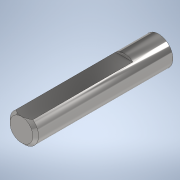
# Autodesk Inventor part: Stepper Motor Shaft
Saved by Autodesk Inventor 2022 (Build 260153000, 153)
## iProperties
Created: 2021-07-23
Part Number: Stepper Motor Shaft
Material: Generic
Document SubType Name: Modeling
Designer: John
Density: 1 g/cm^3
Appearance: Steel - Polished
Author: John
Autodesk Inventor part; units mm, degrees
ref_plane "YZ Plane" through (0, 0, 0) normal (1, 0, 0) x (0, 1, 0)
ref_plane "XZ Plane" through (0, 0, 0) normal (0, 1, 0) x (-1, 0, 0)
ref_plane "XY Plane" through (0, 0, 0) normal (0, 0, 1) x (1, 0, 0)
sketch "Sketch1" plane through (0, 0, 0) normal (0, 0, 1) x (1, 0, 0)
  circle A0 centre (0, 0) radius 2.5
  line L0 (-1.5, 2) -> (1.5, 2)
  dimension "d0" = 5
  constraints: 2 end point, 2 point on circle, 1 centre point, 1 coincident, 1 horizontal
  measures "d0" diameter of A0
sketch "Sketch1 outline for Extrusion1" plane through (0, 0, 0) normal (0, 0, 1) x (1, 0, 0)
  line L0 (1.5, 2) -> (-1.5, 2)
  arc A0 (-1.5, 2) -> (1.5, 2) centre (0, 0) ccw
extrude "Extrusion1" add sketch "Sketch1 outline for Extrusion1" along normal blind 24
sketch "Sketch2" plane through (0, 0, 0) normal (0, 0, -1) x (-1, 0, 0)
  line L0 (-1.5, 2) -> (1.5, 2) projected
  arc A0 (-1.5, 2) -> (1.5, 2) centre (0, 0) ccw projected
  arc A1 (1.5, 2) -> (-1.5, 2) centre (0, 0) ccw
  dimension "d3" = 2.5
  constraints: 2 point on circle, 1 centre point
  measures "d3" radius of A1
sketch "Sketch2 outline for Extrusion2" plane through (0, 0, 0) normal (0, 0, -1) x (-1, 0, 0)
  line L0 (-1.5, 2) -> (1.5, 2)
  arc A0 (1.5, 2) -> (-1.5, 2) centre (0, 0) ccw
extrude "Extrusion2" add sketch "Sketch2 outline for Extrusion2" against normal blind 6
chamfer "Chamfer1" distance 0.5 angle 45 1 edges at (0, -2.5, 24)
body "Solid1"
